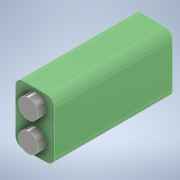
# Autodesk Inventor part: battery
Saved by Autodesk Inventor 2021 (Build 250183000, 183)
## iProperties
Created: 2021-07-13
Part Number: battery
Material: Generic
Document SubType Name: Modeling
Designer: VK
Density: 1 g/cm^3
Appearance: Smooth - Dark Forest Green
Author: VK
Autodesk Inventor part; units mm, degrees
ref_plane "YZ Plane" through (0, 0, 0) normal (1, 0, 0) x (0, 1, 0)
ref_plane "XZ Plane" through (0, 0, 0) normal (0, 1, 0) x (-1, 0, 0)
ref_plane "XY Plane" through (0, 0, 0) normal (0, 0, 1) x (1, 0, 0)
sketch "Sketch1" plane through (0, 0, 0) normal (0, 1, 0) x (-1, 0, 0)
  point P0 (0, 0)
sketch "Sketch2" plane through (0, 0, 0) normal (0, 1, 0) x (-1, 0, 0)
  line L0 (0, 0) -> (10, 0)
  line L1 (10, 0) -> (10, -30)
  line L2 (10, -30) -> (0, -30)
  line L3 (0, -30) -> (0, 0)
  dimension "d0" = 10
  dimension "d1" = 30
  constraints: 8 end point, 2 parallel, 1 horizontal, 1 perpendicular
  measures "d0" distance of L1.end L2.end
  measures "d1" distance of L0.end L1.end
extrude "Extrusion1" add sketch "Sketch2" along normal blind 15
fillet "Fillet1" radius 2 4 edges at (0, 15, -15) (-10, 15, -15) (0, 0, -15) (-10, 0, -15)
sketch "Sketch3" plane through (-8, 0, 0) normal (0, 0, 1) x (1, 0, 0)
  circle A0 centre (3.2708, 11.5209) radius 2.5
  circle A1 centre (3.2708, 4.0226) radius 2.5
  point P0 (8, 0)
  dimension "d5" = 5
  dimension "d6" = 5
  constraints: 2 centre point
  measures "d5" diameter of A0
  measures "d6" diameter of A1
extrude "Extrusion2" add sketch "Sketch3" along normal blind 2
body "Solid1"
